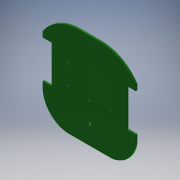
# Autodesk Inventor part: pcb
Saved by Autodesk Inventor 2016 SP1 (Build 200210100, 210)
## iProperties
Created: 2015-03-17
Part Number: pcb
Material: Générique
Document SubType Name: Modeling
Designer: sd
Density: 1 g/cm^3
Appearance: Par défaut
Author: sd
Autodesk Inventor part; units mm, degrees
ref_plane "YZ Plane" through (0, 0, 0) normal (1, 0, 0) x (0, 1, 0)
ref_plane "XZ Plane" through (0, 0, 0) normal (0, 1, 0) x (-1, 0, 0)
ref_plane "XY Plane" through (0, 0, 0) normal (0, 0, 1) x (1, 0, 0)
sketch "Esquisse1" plane through (0, 0, 0) normal (0, 1, 0) x (-1, 0, 0)
  line L0 (-43, -44) -> (43, -44)
  line L1 (43, -44) -> (43, 44)
  line L2 (43, 44) -> (-43, 44)
  line L3 (-43, 44) -> (-43, -44)
  point P0 (0, 0)
  dimension "d0" = 86
  dimension "d1" = 88
  dimension "d2" = 43
  dimension "d3" = 44
  constraints: 8 end point, 2 parallel, 1 horizontal, 1 perpendicular
  measures "d0" distance of L1.end L2.end
  measures "d1" distance of L2.end L0.start
  measures "d2" horizontal distance of point (0, 0) L2.end
  measures "d3" vertical distance of point (0, 0) L2.end
extrude "Carre de base" add sketch "Esquisse1" along normal blind 1.6
sketch "Esquisse2" plane through (0, 1.6, 0) normal (0, 1, 0) x (1, 0, 0)
  line L0 (43, 44) -> (-43, 44) projected
  line L1 (-43, 44) -> (-43, -44) projected
  line L2 (-43, -44) -> (43, -44) projected
  line L3 (43, -44) -> (43, 44) projected
  line L4 (-43, 14) -> (-34.5, 14)
  line L5 (-34.5, 14) -> (-34.5, -21)
  line L6 (-34.5, -21) -> (-43, -21)
  line L7 (43, 14) -> (34.5, 14)
  line L8 (34.5, 14) -> (34.5, -21)
  line L9 (34.5, -21) -> (43, -21)
  line L10 (-43, -21) -> (-43, -26)
  line L11 (43, -21) -> (43, -26)
  line L12 (-43, 14) -> (-43, 19)
  line L13 (43, 14) -> (43, 19)
  line L14 (10, -44) -> (-10, -44)
  line L15 (21, 44) -> (-21, 44)
  arc A0 (10, -44) -> (43, -26) centre (10, -4.75) ccw
  arc A1 (-43, -26) -> (-10, -44) centre (-10, -4.75) ccw
  arc A2 (43, 19) -> (21, 44) centre (17.7955, 19) ccw
  arc A3 (-21, 44) -> (-43, 19) centre (-17.7955, 19) ccw
  point P0 (0, 0)
  dimension "d6" = 35
  dimension "d7" = 30
  dimension "d8" = 30
  dimension "d9" = 8.5
  dimension "d10" = 8.5
  dimension "d11" = 35
  dimension "d13" = 5
  dimension "d14" = 5
  dimension "d15" = 5
  dimension "d16" = 5
  dimension "d21" = 20
  dimension "d22" = 10
  dimension "d23" = 42
  dimension "d24" = 21
  dimension "d25" = 39.25
  dimension "d26" = 39.25
  dimension "d27" = 25.2046
  dimension "d28" = 25.2046
  constraints: 24 end point, 12 point on line, 8 point on circle, 4 centre point, 4 perpendicular, 2 parallel, 2 tangent
  measures "d6" distance of L4.end L5.end
  measures "d7" distance from line of L0 L4.end
  measures "d8" distance between parallel lines of L0 L7
  measures "d9" distance of L7.start L7.end
  measures "d10" distance of L4.start L4.end
  measures "d11" distance of L7.end L8.end
  measures "d13" distance of L9.end L11.end
  measures "d14" distance of L6.end L10.end
  measures "d15" distance of L7.start L13.end
  measures "d16" distance of L4.start L12.end
  measures "d21" distance of L14.start L14.end
  measures "d22" horizontal distance of point (0, 0) L14.start
  measures "d23" distance of L15.start L15.end
  measures "d24" horizontal distance of point (0, 0) L15.start
  measures "d25" radius of A0
  measures "d26" radius of A1
  measures "d27" radius of A2
  measures "d28" radius of A3
extrude "Evidement" cut sketch "Esquisse2" against normal through all contours L3 A2 L0 | A3 L1 L0 | L3 L9 L8 L7 | L4 L5 L6 L1 | L3 L2 A0 | A1 L2 L1
sketch "Esquisse3" plane through (0, 1.6, 0) normal (0, 1, 0) x (1, 0, 0)
  line L0 (34.5, -21) -> (34.5, 14) projected
  line L1 (-34.5, 14) -> (-34.5, -21) projected
  circle A0 centre (-19.5, 5.25) radius 1.05
  circle A1 centre (-19.5, -12.25) radius 1.05
  circle A2 centre (19.5, 5.25) radius 1.05
  circle A3 centre (19.5, -12.25) radius 1.05
  point P0 (0, 0)
  dimension "d31" = 2.1
  dimension "d32" = 17.5
  dimension "d33" = 2.1
  dimension "d34" = 2.1
  dimension "d35" = 2.1
  dimension "d36" = 17.5
  dimension "d37" = 15
  dimension "d38" = 15
  dimension "d39" = 15
  dimension "d40" = 15
  dimension "d41" = 35
  dimension "d42" = 8.75
  dimension "d43" = 8.75
  constraints: 4 centre point
  measures "d31" diameter of A0
  measures "d32" distance of A3.centre A2.centre
  measures "d33" diameter of A1
  measures "d34" diameter of A3
  measures "d35" diameter of A2
  measures "d36" distance of A1.centre A0.centre
  measures "d37" distance from line of L0 A2.centre
  measures "d38" distance from line of L0 A3.centre
  measures "d39" distance from line of L1 A0.centre
  measures "d40" distance from line of L1 A1.centre
  measures "d41" distance of L1.start L1.end
  measures "d42" vertical distance of A0.centre L1.start
  measures "d43" vertical distance of A2.centre L0.end
extrude "Extrusion4" cut sketch "Esquisse3" against normal through all
sketch "Esquisse4" plane through (0, 1.6, 0) normal (0, 1, 0) x (1, 0, 0)
  line L0 (21, 44) -> (-21, 44) projected
  circle A0 centre (0, 26.5) radius 1.5
  line L1 (43, 14) -> (43, 19) projected
  line L2 (-43, 19) -> (-43, 14) projected
  point P0 (0, 0)
  dimension "d46" = 3
  dimension "d47" = 17.5
  dimension "d57" = 86
  dimension "d58" = 43
  constraints: 1 centre point
  measures "d46" diameter of A0
  measures "d47" distance from line of L0 A0.centre
  measures "d57" distance between parallel lines of L1 L2
  measures "d58" distance from line of L2 A0.centre
extrude "Extrusion5" cut sketch "Esquisse4" against normal through all
sketch "Esquisse5" plane through (0, 0, 0) normal (0, -1, 0) x (1, 0, 0)
  line L0 (-43, -19) -> (-43, -14) projected
  line L1 (21, -44) -> (-21, -44) projected
  line L2 (43, -14) -> (43, -19) projected
  circle A0 centre (0, -7.5) radius 1.25
  point P0 (0, 0)
  dimension "d51" = 2.5
  dimension "d52" = 36.5
  dimension "d53" = 43
  dimension "d54" = 86
  constraints: 1 centre point
  measures "d51" diameter of A0
  measures "d52" distance from line of L1 A0.centre
  measures "d53" distance from line of L0 A0.centre
  measures "d54" distance between parallel lines of L2 L0
extrude "Extrusion6" cut sketch "Esquisse5" against normal through all
equation "\"d2\" = 0.5 * d0"
equation "\"d3\" = 0.5 * d1"
equation "\"d8\" = d7"
equation "\"d9\" = d10"
equation "\"d11\" = d6"
equation "\"d13\" = d14"
equation "\"d15\" = d16"
equation "\"d22\" = 0.5 * d21"
equation "\"d24\" = 0.5 * d23"
equation "\"d26\" = d25"
equation "\"d28\" = d27"
equation "\"d33\" = d31"
equation "\"d34\" = d31"
equation "\"d35\" = d31"
equation "\"d36\" = d32"
equation "\"d38\" = d37"
equation "\"d39\" = d37"
equation "\"d40\" = d37"
equation "\"d42\" = -0.5 * d36 + 0.5 * d41"
equation "\"d43\" = d42"
equation "\"d58\" = 0.5 * d57"
equation "\"d53\" = 0.5 * d54"
